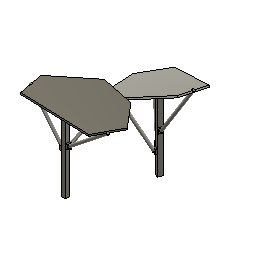
monorail-multi (Autodesk Fusion 360 design; units mm, degrees)
Autodesk Fusion 360 part; units mm, degrees
sketch "Sketch1" plane through (0, 0, 0) normal (0, 1, 0) x (1, 0, 0) in component "monorail v4"
  line L0 (0, 0) -> (-5, 0)
  line L1 (-5, 0) -> (-5, -5)
  line L2 (-5, -5) -> (0, -5)
  line L3 (0, -5) -> (0, 0)
  constraint horizontal L0
  constraint vertical L1
  constraint horizontal L2
  constraint vertical L3
  constraint coincident L0.start L3.end
extrude "Extrude1" add sketch "Sketch1" along normal blind 2.5 makes body 1 in component "monorail v4"
extrude "Extrude2" add 1 faces at (-3.3333, 2.5, 1.6667) along direction (0, 1, 0) blind 80 on bodies 1 bodies 1 in component "monorail v4"
sketch "Sketch2" plane through (0, 0, 0) normal (0, 0, 1) x (1, 0, 0) in component "monorail v4"
  line L0 (0, 5) -> (2, 5)
  line L1 (2, 5) -> (2, 10)
  line L2 (2, 10) -> (0, 10)
  line L3 (0, 10) -> (0, 5)
  constraint horizontal L0
  constraint vertical L1
  constraint horizontal L2
  constraint vertical L3
extrude "Extrude3" add sketch "Sketch2" along normal blind 5 separate body makes body 2 in component "monorail v4"
sphere "SpherePrimitive1" cut diameter 2.5 placed x (0, 0, -1) y (0, 1, 0) z (1, 0, 0) at (2, 7.5, 2.5) bodies 2 in component "monorail v4"
cylinder "CylinderPrimitive1" add diameter 3.5 height 45 placed x (1, 0, 0) y (0, 0, -1) z (0, 1, 0) at (15, 0, 0) separate body makes body 3 in component "monorail v4"
extrude "Extrude4" add 1 faces at (14.4232, 45, -0.7066) along direction (0, 1, 0) blind 15 on bodies 3 bodies 3 in component "monorail v4"
sphere "SpherePrimitive2" add diameter 2.5 placed x (1, 0, 0) y (0, 0, 1) z (0, -1, 0) at (15, 0, 0) bodies 3 in component "monorail v4"
sphere "SpherePrimitive3" add diameter 2.5 placed x (-1, 0, 0) y (0, 0, 1) z (0, 1, 0) at (15, 60, 0) bodies 3 in component "monorail v4"
copy_body "CopyPasteBodies1" bodies 3 2 makes body 4 makes body 5 in component "monorail v4"
move_body "Move1" bodies 4 5 to x (1, 0, 0) y (0, 1, 0) z (0, 0, 1) at (-12.4926, 0, -17.6032) in component "monorail v4"
copy_body "CopyPasteBodies3" bodies 4 makes body 6 in component "monorail v4"
move_body "Move2" bodies 6 to x (1, 0, 0) y (0, 1, 0) z (0, 0, 1) at (19.3713, 0, -0.932) in component "monorail v4"
copy_body "CopyPasteBodies4" bodies 5 makes body 7 in component "monorail v4"
move_body "Move3" bodies 7 to x (1, 0, 0) y (0, 1, 0) z (0, 0, 1) at (-10.1487, 0, 0) in component "monorail v4"
sketch "Sketch9" plane through (0, 0, 0) normal (0, 1, 0) x (1, 0, 0) in component "monorail v4"
  line L0 (20, 0) -> (0, -25)
  line L1 (0, -25) -> (-22.7284, 8.4291)
  line L2 (-22.7284, 8.4291) -> (20, 0)
  line L3 (11.59, -26.3409) -> (26.0343, -8.2855)
  line L4 (26.0343, -8.2855) -> (16.8582, 12.7941)
  line L5 (16.8582, 12.7941) -> (-32.8132, 15.2024)
  line L6 (-32.8132, 15.2024) -> (-36.4257, -4.8166)
  line L7 (-36.4257, -4.8166) -> (-12.0415, -29.8028)
  line L8 (-12.0415, -29.8028) -> (11.59, -26.3409)
  constraint parallel L0 L3
extrude "Extrude5" add sketch "Sketch9" along normal blind 2 separate body contours L0 L1 L2 | L3 L4 L5 L6 L7 L8 makes body 8 in component "monorail v4"
move_body "Move4" bodies 8 to x (1, 0, 0) y (0, 1, 0) z (0, 0, 1) at (0, 105.9344, 0) in component "monorail v4"
scale "Scale1" factor 1.5 about (-36.4257, 107.9344, 4.8166) bodies 8 in component "monorail v4"
extrude "Extrude6" cut 1 faces at (2.4083, 107.9344, 8.5043) along direction (0, -1, 0) blind 1 on bodies 8 bodies 8 in component "monorail v4"
copy_body "Body->Comp1" bodies 3 removing the originals makes body 9 in component "poleLeft"
copy_body "Body->Comp2" bodies 8 removing the originals makes body 10 in component "FLAT"
copy_body "Body->Comp3" bodies 4 removing the originals makes body 11 in component "poleRight"
copy_body "Body->Comp4" bodies 5 removing the originals makes body 12 in component "gantryRight"
copy_body "Body->Comp5" bodies 2 removing the originals makes body 13 in component "gantryLeft"
copy_body "Body->Comp6" bodies 1 removing the originals makes body 14 in component "mainHole"
copy_body "Body->Comp7" bodies 7 removing the originals makes body 15 in component "gantryBack"
copy_body "Body->Comp8" bodies 6 removing the originals makes body 16 in component "poleBack"
sketch "Sketch1 (2)" plane through (0, 0, 0) normal (0, 0, 1) x (1, 0, 0)
component "monorail v4" placed x (1, 0, 0) y (0, 1, 0) z (0, 0, 1) at (0, 0, 0)
component "monorail v4" placed x (-0.911886, 0, -0.410443) y (0, 1, 0) z (0.410443, 0, -0.911886) at (26.8044, 0, -72.7232)
component "poleLeft" placed x (0.92689, -0.039778, 0.373219) y (0.253175, 0.800345, -0.543461) z (-0.277087, 0.598218, 0.751903) at (-16.4034, 32.5038, -7.5983) in component "monorail v4"
component "FLAT" placed x (0.932722, -0.360428, -0.011048) y (-0.359446, -0.931753, 0.05133) z (-0.028795, -0.043906, -0.998621) at (35.5992, 187.7497, -0.2544) in component "monorail v4"
component "poleRight" placed x (-0.521098, -0.046881, -0.852208) y (-0.437889, 0.871746, 0.2198) z (0.732605, 0.48771, -0.474794) at (7.2028, 58.9748, -3.7211) in component "monorail v4"
component "gantryRight" placed x (0, 0, -1) y (0, 1, 0) z (1, 0, 0) at (12.6032, 24.4072, -12.4926) in component "monorail v4"
component "gantryLeft" placed x (1, 0, 0) y (0, -1, 0) z (0, 0, -1) at (0, 35.9285, 5) in component "monorail v4"
component "mainHole" placed x (1, 0, 0) y (0, 1, 0) z (0, 0, 1) at (0, 0, 0) in component "monorail v4"
component "gantryBack" placed x (-1, 0, 0) y (0, -1, 0) z (0, 0, 1) at (-27.6413, 57.772, 17.6032) in component "monorail v4"
component "poleBack" placed x (0.617372, -0.695433, 0.36773) y (0.705355, 0.69633, 0.132662) z (-0.348319, 0.177478, 0.920421) at (-17.9634, 46.9332, 11.5147) in component "monorail v4"
named bodies: "mainHole", "gantryLeft", "poleLeft", "poleRight", "gantryRight", "poleBack", "gantryBack", "FLAT"
